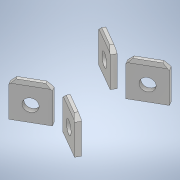
# Autodesk Inventor part: contact
Saved by Autodesk Inventor 2022.1 (Build 261234000, 234)
## iProperties
Created: 2019-08-22
Part Number: contact
Material: Нержавеющая сталь
Document SubType Name: Modeling
Designer: Иванов Д.А.
Mass: 1.21016 g
Surface Area: 4.34284 cm^2
Volume: 0.15127 cm^3
Density: 8 g/cm^3
Appearance: С умеренной полировкой
Author: Иванов Д.А.
Autodesk Inventor part; units mm, degrees
ref_plane "YZ Plane" through (0, 0, 0) normal (1, 0, 0) x (0, 1, 0)
ref_plane "XZ Plane" through (0, 0, 0) normal (0, 1, 0) x (-1, 0, 0)
ref_plane "XY Plane" through (0, 0, 0) normal (0, 0, 1) x (1, 0, 0)
sketch "Эскиз1" plane through (0, 0, 0) normal (0, 0, 1) x (1, 0, 0)
  arc A0 (3.0397, -11.35) -> (11.3865, -2.9) centre (0, 0) ccw projected
  arc A1 (-3.0397, 11.35) -> (-3.0397, -11.35) centre (0, 0) ccw projected
  arc A2 (11.3865, 2.9) -> (3.0397, 11.35) centre (0, 0) ccw projected
  line L0 (0, 11.5515) -> (0, -11.5515) construction
  line L1 (-11.75, 0) -> (11.75, 0) construction
  line L2 (6.5493, 9.608) -> (7.0493, 8.742)
  line L3 (7.0493, 8.742) -> (1.55, 5.567)
  line L4 (1.55, 5.567) -> (1.05, 6.433)
  line L5 (1.05, 6.433) -> (6.5493, 9.608)
  line L6 (6.7993, 9.175) -> (1.3, 6) construction
  point P0 (0, 0)
  point P1 (0, 0)
  dimension "d0" = 1
  dimension "d1" = 6.35
  dimension "d2" = 30
  dimension "d3" = 12
  dimension "d4" = 2.6
  constraints: 14 end point, 4 midpoint, 2 perpendicular, 1 coincident, 1 point on circle
  measures "d0" distance between parallel lines of L3 L5
  measures "d1" distance between parallel lines of L4 L2
  measures "d2" angle of L1 L6
  measures "d3" diameter of L6.end L1
  measures "d4" diameter of L6.end L0
extrude "Выдавливание1" add sketch "Эскиз1" along normal blind 7
chamfer "Фаска1" distance 0.2 angle 75 2 edges at (4.2996, 7.1545, 7) (3.7996, 8.0205, 7) measured on face at (5.0495, 7.9723, 7)
chamfer "Фаска2" distance 1 angle 45 2 edges at (1.3, 6, 7) (6.7993, 9.175, 7)
sketch "Эскиз2" plane through (1.55, 5.567, 0) normal (0.5, -0.8660254, 0) x (0.8660254, 0.5, 0)
  circle A0 centre (3.175, 3) radius 1.25
  line L0 (5.35, 7) -> (1, 7) projected
  line L1 (6.35, 0) -> (0, 0) projected
  line L2 (3.175, 7) -> (3.175, 0) construction
  point P0 (-4.1258, 0)
  dimension "d13" = 2.5
  dimension "d14" = 4
  constraints: 2 end point, 2 midpoint, 1 centre point, 1 point on line
  measures "d13" diameter of A0
  measures "d14" distance from line of A0.centre L0
extrude "Выдавливание2" cut sketch "Эскиз2" against normal up to next
pattern_circular "Круговой массив1" count 2 over 360 about axis through (0, 0, -10) along (0, 0, 1) of "Выдавливание1", "Фаска1", "Фаска2", "Выдавливание2"
mirror "Зеркальное отражение1" about plane through (0, 0, 0) normal (1, 0, 0) of "Выдавливание1", "Фаска1", "Фаска2", "Выдавливание2", "Круговой массив1"
